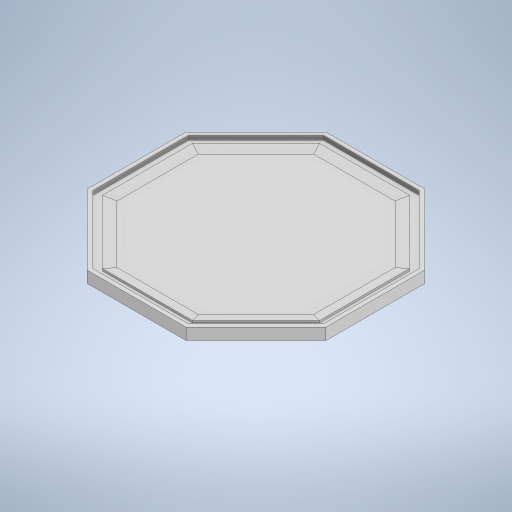
# Autodesk Inventor part: OV-PAM_bottom_2
Saved by Autodesk Inventor 2024 (Build 280153000, 153)
## iProperties
Created: 2023-06-16
Part Number: OV-PAM_bottom_2
Material: 일반
Document SubType Name: Modeling
Designer: jsw
Density: 1 g/cm^3
Appearance: 기본값
Author: jsw
Autodesk Inventor part; units mm, degrees
ref_plane "YZ Plane" through (0, 0, 0) normal (1, 0, 0) x (0, 1, 0)
ref_plane "XZ Plane" through (0, 0, 0) normal (0, 1, 0) x (-1, 0, 0)
ref_plane "XY Plane" through (0, 0, 0) normal (0, 0, 1) x (1, 0, 0)
sketch "스케치3" plane through (0, 0, 0) normal (0, 1, 0) x (-1, 0, 0)
  line L0 (34.9919, -14.4941) -> (14.4941, -34.9919)
  line L1 (14.4941, -34.9919) -> (-14.4941, -34.9919)
  line L2 (-14.4941, -34.9919) -> (-34.9919, -14.4941)
  line L3 (-34.9919, -14.4941) -> (-34.9919, 14.4941)
  line L4 (-34.9919, 14.4941) -> (-14.4941, 34.9919)
  line L5 (-14.4941, 34.9919) -> (14.4941, 34.9919)
  line L6 (14.4941, 34.9919) -> (34.9919, 14.4941)
  line L7 (34.9919, 14.4941) -> (34.9919, -14.4941)
  line L8 (13.5, -32.5919) -> (-13.5, -32.5919)
  line L9 (-13.5, -32.5919) -> (-32.5919, -13.5)
  line L10 (-32.5919, -13.5) -> (-32.5919, 13.5)
  line L11 (-32.5919, 13.5) -> (-13.5, 32.5919)
  line L12 (-13.5, 32.5919) -> (13.5, 32.5919)
  line L13 (13.5, 32.5919) -> (32.5919, 13.5)
  line L14 (32.5919, 13.5) -> (32.5919, -13.5)
  line L15 (32.5919, -13.5) -> (13.5, -32.5919)
  point P0 (0, 0)
  point P1 (0, 0)
  point P2 (0, 0)
  point P3 (0, 0)
  dimension "d66" = 27
  dimension "d67" = 2.4
  constraints: 32 end point, 3 coincident, 2 horizontal, 34 other
  measures "d66" distance of L8.start L8.end
  measures "d67" distance between parallel lines of L15 L0
extrude "돌출2" add sketch "스케치3" along normal blind 3.4 contours L0 L1 L2 L3 L4 L5 L6 L7 | L8 L9 L10 L11 L12 L13 L14 L15
sketch "스케치4" plane through (0, 3.4, 0) normal (0, 1, 0) x (1, 0, 0)
  line L0 (13.5, -32.5919) -> (-13.5, -32.5919)
  line L1 (-13.5, -32.5919) -> (-32.5919, -13.5)
  line L2 (-32.5919, -13.5) -> (-32.5919, 13.5)
  line L3 (-32.5919, 13.5) -> (-13.5, 32.5919)
  line L4 (-13.5, 32.5919) -> (13.5, 32.5919)
  line L5 (13.5, 32.5919) -> (32.5919, 13.5)
  line L6 (32.5919, 13.5) -> (32.5919, -13.5)
  line L7 (32.5919, -13.5) -> (13.5, -32.5919)
  line L8 (-13.9971, 33.7919) -> (13.9971, 33.7919)
  line L9 (13.9971, 33.7919) -> (33.7919, 13.9971)
  line L10 (33.7919, 13.9971) -> (33.7919, -13.9971)
  line L11 (33.7919, -13.9971) -> (13.9971, -33.7919)
  line L12 (13.9971, -33.7919) -> (-13.9971, -33.7919)
  line L13 (-13.9971, -33.7919) -> (-33.7919, -13.9971)
  line L14 (-33.7919, -13.9971) -> (-33.7919, 13.9971)
  line L15 (-33.7919, 13.9971) -> (-13.9971, 33.7919)
  line L16 (-13.1686, 31.7919) -> (13.1686, 31.7919)
  line L17 (13.1686, 31.7919) -> (31.7919, 13.1686)
  line L18 (31.7919, 13.1686) -> (31.7919, -13.1686)
  line L19 (31.7919, -13.1686) -> (13.1686, -31.7919)
  line L20 (13.1686, -31.7919) -> (-13.1686, -31.7919)
  line L21 (-13.1686, -31.7919) -> (-31.7919, -13.1686)
  line L22 (-31.7919, -13.1686) -> (-31.7919, 13.1686)
  line L23 (-31.7919, 13.1686) -> (-13.1686, 31.7919)
  point P0 (0, 0)
  point P1 (0, 0)
  point P2 (0, 0)
  point P3 (0, 0)
  dimension "d7" = 27
  dimension "d68" = 1.2
  dimension "d69" = 0.8
  constraints: 48 end point, 3 coincident, 3 horizontal, 51 other
  measures "d7" distance of L1.end L2.end
  measures "d68" distance between parallel lines of L3 L15
  measures "d69" distance between parallel lines of L16 L4
extrude "돌출3" cut sketch "스케치4" against normal blind 1.2 contours L0 L1 L2 L3 L4 L5 L6 L7 | L8 L9 L10 L11 L12 L13 L14 L15 | L16 L17 L18 L19 L20 L21 L22 L23
sketch "스케치9" plane through (0, 0, 0) normal (0, -1, 0) x (1, 0, 0)
  line L0 (7.5, 10) -> (2.5, 10)
  line L1 (2.5, 10) -> (2.5, -10)
  line L2 (2.5, -10) -> (7.5, -10)
  line L3 (7.5, -10) -> (7.5, 10)
  line L4 (7.5, 10) -> (2.5, -10) construction
  line L5 (2.5, 10) -> (7.5, -10) construction
  line L6 (-2.5, 10) -> (-7.5, 10)
  line L7 (-7.5, 10) -> (-7.5, -10)
  line L8 (-7.5, -10) -> (-2.5, -10)
  line L9 (-2.5, 10) -> (-7.5, -10) construction
  line L10 (-7.5, 10) -> (-2.5, -10) construction
  line L11 (-2.5, -10) -> (-2.5, 10)
  point P0 (0, 0)
  point P1 (5, 0)
  point P2 (-5, 0)
  dimension "d42" = 20
  dimension "d43" = 5
  dimension "d44" = 2.5
  dimension "d47" = 10
  constraints: 24 end point, 2 horizontal, 2 midpoint, 2 parallel, 1 collinear, 1 horizontal alignment, 1 perpendicular, 10 other
  measures "d42" distance of L2.end L0.start
  measures "d43" distance of L1.end L2.end
  measures "d44" distance from line of L1 point (0, 0)
  measures "d47" distance of L0.start L6.start
extrude "돌출8" add sketch "스케치9" along normal blind 10
sketch "스케치10" plane through (-7.5, 0, -10) normal (-1, 0, 0) x (0, 0, 1)
  circle A0 centre (15, -5) radius 1.25
  line L0 (19.9591, 0) -> (0.0886, 0)
  line L1 (24.4941, 0) -> (-4.4941, 0) projected
  circle A1 centre (5, -5) radius 1.25
  line L2 (20, 0) -> (20, -10) projected
  point P0 (10, 0)
  dimension "d54" = 2.5
  dimension "d57" = 10
  dimension "d62" = 5
  dimension "d63" = 5
  constraints: 2 centre point, 2 end point, 1 horizontal, 1 point on line, 2 other
  measures "d54" diameter of A0
  measures "d57" distance of A0.centre A1.centre
  measures "d62" distance from line of L0 A0.centre
  measures "d63" distance from line of L2 A0.centre
extrude "돌출9" cut sketch "스케치10" against normal blind 20
sketch "스케치11" plane through (0, 2.2, 0) normal (0, 1, 0) x (1, 0, 0)
  line L0 (-13.1686, 31.7919) -> (13.1686, 31.7919)
  line L1 (13.1686, 31.7919) -> (31.7919, 13.1686)
  line L2 (31.7919, 13.1686) -> (31.7919, -13.1686)
  line L3 (31.7919, -13.1686) -> (13.1686, -31.7919)
  line L4 (13.1686, -31.7919) -> (-13.1686, -31.7919)
  line L5 (-13.1686, -31.7919) -> (-31.7919, -13.1686)
  line L6 (-31.7919, -13.1686) -> (-31.7919, 13.1686)
  line L7 (-31.7919, 13.1686) -> (-13.1686, 31.7919)
  line L8 (-13.9971, 33.7919) -> (13.9971, 33.7919) projected
  line L9 (-11.926, 28.7919) -> (11.926, 28.7919)
  line L10 (11.926, 28.7919) -> (28.7919, 11.926)
  line L11 (28.7919, 11.926) -> (28.7919, -11.926)
  line L12 (28.7919, -11.926) -> (11.926, -28.7919)
  line L13 (11.926, -28.7919) -> (-11.926, -28.7919)
  line L14 (-11.926, -28.7919) -> (-28.7919, -11.926)
  line L15 (-28.7919, -11.926) -> (-28.7919, 11.926)
  line L16 (-28.7919, 11.926) -> (-11.926, 28.7919)
  point P0 (0, 0)
  point P1 (0, 0)
  point P2 (0, 0)
  dimension "d70" = 2
  dimension "d71" = 3
  constraints: 32 end point, 2 coincident, 2 horizontal, 34 other
  measures "d70" distance between parallel lines of L8 L0
  measures "d71" distance between parallel lines of L9 L0
extrude "돌출10" add sketch "스케치11" along normal blind 0.6
chamfer "모따기1" distance 3 distance2 0.6 1 edges at (-28.7919, 2.8, 0) measured on face at (-29.2919, 2.8, 0)
chamfer "모따기2" distance 3 distance2 0.6 2 edges at (-30.2918, 2.8, -10.426) (-20.3589, 2.8, -20.3589) measured on face at (-20.7125, 2.8, -20.7125) measured on face at (-30.6454, 2.8, -10.7796)
chamfer "모따기3" distance 3 distance2 0.6 2 edges at (-14.0472, 2.8, -28.7919) (0, 2.8, -28.7919) measured on face at (-14.0472, 2.8, -29.2919) measured on face at (0, 2.8, -29.2919)
chamfer "모따기4" distance 3 distance2 0.6 2 edges at (10.426, 2.8, -30.2918) (20.3589, 2.8, -20.3589) measured on face at (10.7796, 2.8, -30.6454) measured on face at (20.7125, 2.8, -20.7125)
chamfer "모따기5" distance 3 distance2 0.6 2 edges at (28.7919, 2.8, -14.0472) (28.7919, 2.8, 0) measured on face at (29.2919, 2.8, 0) measured on face at (29.2919, 2.8, -14.0472)
chamfer "모따기6" distance 3 distance2 0.6 2 edges at (30.2918, 2.8, 10.426) (20.3589, 2.8, 20.3589) measured on face at (30.6454, 2.8, 10.7796) measured on face at (20.7125, 2.8, 20.7125)
chamfer "모따기7" distance 3 distance2 0.6 2 edges at (14.0472, 2.8, 28.7919) (0, 2.8, 28.7919) measured on face at (0, 2.8, 29.2919) measured on face at (14.0472, 2.8, 29.2919)
chamfer "모따기8" distance 3 distance2 0.6 3 edges at (-10.426, 2.8, 30.2918) (-20.3589, 2.8, 20.3589) (-30.2918, 2.8, 10.426) measured on face at (-20.7125, 2.8, 20.7125) measured on face at (-10.7796, 2.8, 30.6454) measured on face at (-30.6454, 2.8, 10.7796)
